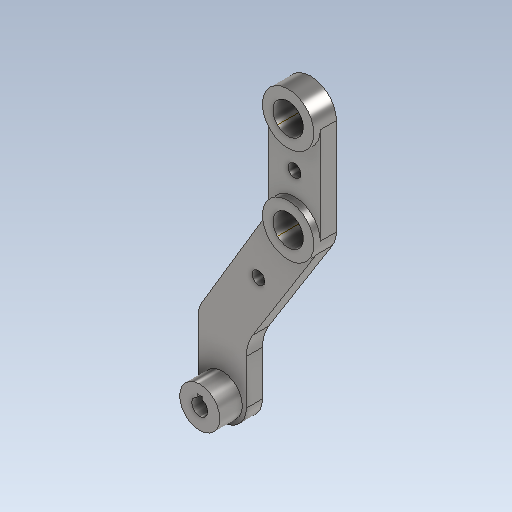
# Autodesk Inventor part: ParallelSystem_ProximalPart_Driven_Counterpart_v2.1_AxialNadellager
Saved by Autodesk Inventor 2022 (Build 260153000, 153)
## iProperties
Created: 2022-07-18
Part Number: ParallelSystem_ProximalPart_Driven_Counterpart_v2.1_AxialNadellager
Material: Edelstahl
Document SubType Name: Modeling
Designer: alexw
Density: 8 g/cm^3
Appearance: Halbpoliert
Mass: 237.14 g
Surface Area: 170.01 cm^2
Volume: 29.6426 cm^3
d0: 10,000 mm
d1: 25,000 mm
d4: 30,000 mm
d7: 5,000 mm
d8: 0,00 grd
d9: 6,000 mm
d10: 0,00 grd
d11: 25,000 mm
d23: 8,000 mm
d36: 0,00 grd
d37: 30,000 mm
d38: 60,00 grd
d39: 35,000 mm
d40: 90,000 mm
d41: 60,000 mm
d42: 45,000 mm
d43: 19,000 mm
d44: 12,000 mm
d45: 30,000 mm
Passfeder_width: 3,000 mm
Nabennuttiefe: 1,400 mm
d51: 3,000 mm
d52: 1,400 mm
ParallelLink_BearingStep_Height: 10,000 mm
ParallelLink_Lever_Thickness: 14,000 mm
ParallelHebel_Gabelgelenk_OuterDia: 32,000 mm
Nadellager_OuterDia: 19,000 mm
ParallelHebel_Passflansch_HoleDia: 25,500 mm
Author: alexw
Autodesk Inventor part; units mm, degrees
ref_plane "YZ Plane" through (0, 0, 0) normal (1, 0, 0) x (0, 1, 0)
ref_plane "XZ Plane" through (0, 0, 0) normal (0, 1, 0) x (-1, 0, 0)
ref_plane "XY Plane" through (0, 0, 0) normal (0, 0, 1) x (1, 0, 0)
sketch "Skizze1" plane through (0, 0, 0) normal (0, 0, 1) x (1, 0, 0)
  arc A0 (-1.5, 4.7697) -> (1.5, 4.7697) centre (0, 0) ccw
  circle A1 centre (0, 0) radius 12.5
  line L0 (-30.9429, 0) -> (77.0229, 0) construction
  circle A2 centre (0, 0) radius 15
  circle A3 centre (45, 112.9423) radius 16
  line L1 (61, 112.9423) -> (61, 172.9423)
  line L2 (29, 112.9423) -> (29, 172.9423)
  line L3 (45, 112.9423) -> (45, 188.9423) construction
  line L4 (45, 112.9423) -> (45, 128.9423) construction
  line L5 (29, 112.9423) -> (61, 112.9423) construction
  line L6 (-15, 0) -> (-15, 35)
  line L7 (15, 0) -> (15, 35)
  line L8 (-15, 35) -> (15, 35) construction
  circle A4 centre (0, 35) radius 15 construction
  line L9 (-12.8844, 42.6807) -> (29, 112.9423)
  arc A5 (-12.8844, 42.6807) -> (-15, 35) centre (0, 35) ccw
  line L10 (15, 35) -> (58.5544, 104.4407)
  arc A6 (58.5544, 104.4407) -> (61, 112.9423) centre (45, 112.9423) ccw
  line L11 (0, 35) -> (45, 112.9423) construction
  circle A7 centre (45, 172.9423) radius 16
  circle A8 centre (45, 172.9423) radius 9.5
  circle A9 centre (45, 112.9423) radius 9.5
  line L12 (-1.5, 6.4) -> (1.5, 6.4)
  line L13 (1.5, 6.4) -> (1.5, 4.7697)
  line L14 (-1.5, 4.7697) -> (-1.5, 6.4)
  line L15 (0, 0) -> (0, 5) construction
  line L16 (0, 5) -> (1.5, 5) construction
  circle A10 centre (45, 112.9423) radius 12.75 construction
  circle A11 centre (45, 172.9423) radius 12.75 construction
  point P0 (22.5, 73.9711)
  point P1 (45, 142.9423)
  point P2 (-13, 0)
  point P3 (13, 0)
  point P4 (0, 6.4)
  point P5 (45, 125.6923)
  point P6 (33.9582, 106.5673)
  point P7 (56.0418, 106.5673)
  point P8 (45, 185.6923)
  point P9 (33.9582, 166.5673)
  point P10 (56.0418, 166.5673)
  dimension "d69" = 25.5
  dimension "ParallelHebel_Passflansch_HoleDia" = 25.5
  dimension "d0" = 10
  dimension "d1" = 25
  dimension "d4" = 30
  dimension "d36" = 0
  dimension "ParallelHebel_Gabelgelenk_OuterDia" = 32
  dimension "d38" = 60
  dimension "d39" = 35
  dimension "d40" = 90
  dimension "d41" = 60
  dimension "d42" = 45
  dimension "d43" = 19
  dimension "Nadellager_OuterDia" = 19
  dimension "d45" = 30
  dimension "d51" = 3
  dimension "d52" = 1.4
  dimension "d67" = 360
  dimension "d72" = 360
  constraints: 32 end point, 17 point on circle, 13 tangent, 10 centre point, 10 point on line, 8 coincident, 5 perpendicular, 4 midpoint, 2 equal radius, 2 horizontal, 2 parallel, 2 vertical, 2 vertical alignment, 12 other
  measures "d0" diameter of A0
  measures "d1" diameter of A1
  measures "d4" diameter of A2
  measures "d36" distance between parallel lines of L3 L4
  measures "ParallelHebel_Gabelgelenk_OuterDia" diameter of A3
  measures "d38" angle of L8 L11
  measures "d39" distance of A4.centre point (0, 0)
  measures "d40" distance of point (45, 112.942) A4.centre
  measures "d41" distance of A7.centre point (45, 112.942)
  measures "d42" distance of point (22.5, 73.971) A4.centre
  measures "d43" diameter of A8
  measures "Nadellager_OuterDia" diameter of A9
  measures "d45" distance of point (45, 142.942) point (45, 112.942)
  measures "d51" distance of L12.start L12.end
  measures "d52" distance between parallel lines of L12 L16
extrude "Extrusion1" add sketch "Skizze1" along normal blind 10 contours A1
extrude "Extrusion2" add sketch "Skizze1" against normal blind 14 contours A1 | A2 | A2 L6 A5 L9 A3 L10 L7 | A3 | L2 A7 L1 A3 | A7
extrude "Extrusion4" cut sketch "Skizze1" against normal blind 4 contours A2 | A2 L6 A5 L9 A3 L10 L7 | L2 A7 L1 A3
fillet "Rundung1" radius 25 2 edges at (29, 112.9423, -9) (15, 35, -9)
hole "Bohrung2" at (45, 142.9423, 0) at (22.5, 73.9711, 0) direction (0, 0, -1) diameter 8 end through all
ref_plane "Arbeitsebene1" through (45, 112.9423, 0) normal (1, 0, 0) x (0, 0, -1)
